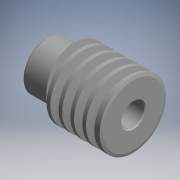
# Autodesk Inventor part: SW2-R1_On
Saved by Autodesk Inventor 2017.3 (Build 213256000, 256)
## iProperties
Part Number: SW2-R1_On
Material: Generic
Catalog Web Link: www.cadenas.de
Description: Worms, Worm Gears (SW)1-
Vendor: KHK
Document SubType Name: Modeling
Designer: partserver
Manufacturer: KHK
Mass: 24.6857 g
Surface Area: 108.891 cm^2
Volume: 24.6857 cm^3
Density: 1 g/cm^3
Appearance: PSOLRGB-192-192-192
Category: PARTsolutions
Company: KHK
Title: SW2-R1
Author: Cadenas PARTsolutions
PSOL_IDENT_0: {$CADENAS_DATA\23d-libs\khk\worms_worms_gears\ww_gears_sw.prj},178 {VTYP=3D},{NB=SW2-R1_On},{LINA=SW
PSOL_IDENT_1: 2-R1},{NN=Worms, Worm Gears (SW)1},{DATE=10.04.2020 06:07:44},{GEOMDATE=25.03.2019 13:28:29},{VERSIO
PSOL_IDENT_2: N=},{LINEID=120},{WBVAR=TOOTH},{WBNUMERIC=}  {NB=SW2-R1_On},{LINA=SW2-R1},{KT=DUMMY},{CN=SW2-R1},{NM=
PSOL_IDENT_3: 2.00},{NS=1},{LA=3.70},{HT=R},{SH=W1},{L=12},{M=25},{N=31},{O=35},{P=32},{Q=14},{Q1=0},{R=46},{K=0},
PSOL_IDENT_4: {KD=0.0},{SCS=0},{S=0},{WMF=W1002.WMF},{NDM=0},{KDM=0.000},{X=0.5},{Y=0.5},{H1=16.000},{AN=14.931},{
PSOL_IDENT_5: U=16},{COM1=1,'Only selection gear',201,'BG2-20R1',20,'CG2-20R1',30,'CG2-30R1',40,'CG2-40R1',50,'CG2
PSOL_IDENT_6: -50R1'},{XX=1},{TOOTH=On},{POINT=2.200}
NB: SW2-R1_On
NN: Worms, Worm Gears (SW)1
NBSYN: $CN._$TOOTH.
LINA: SW2-R1
CATALOG: KHK
CN: SW2-R1
NM: 2
NS: 1
LA: 3.7
HT: R
SH: W1
L: 12
M: 25
N: 31
O: 35
P: 32
Q: 14
Q1: 0
R: 46
K: 0
KD: 0
SCS: 0
S: 0
TOOTH: On
POINT: 2.2
SUPPLIER: KHK
ARTICLENO: SW2-R1_On
BOMINFO: SW2-R1
CREATOR: CADENAS GmbH
Autodesk Inventor part; units mm, degrees
sketch "Sketch_1" plane through (0, 0, 0) normal (0, 0, 1) x (1, 0, 0)
  line L0 (46, 0) -> (0, 0)
  line L1 (0, 6.5) -> (0.5, 6)
  line L2 (0.5, 6) -> (45.5, 6)
  line L3 (45.5, 6) -> (46, 6.5)
  line L4 (46, 6.5) -> (46, 12)
  line L5 (46, 12) -> (45.5, 12.5)
  line L6 (45.5, 12.5) -> (32, 12.5)
  line L7 (32, 12.5) -> (32, 16)
  line L8 (32, 16) -> (31.6, 17.5)
  line L9 (31.6, 17.5) -> (0.4, 17.5)
  line L10 (0.4, 17.5) -> (0, 16)
  line L11 (0, 16) -> (0, 6.5)
  constraints: 24 end point
revolve "Revolution1" add sketch "Sketch_1" angle 360 about axis through (46, 0, 0) along (1, 0, 0)
sketch "Sketch_18" plane through (0, 0, 0) normal (0, 0, 1) x (1, 0, 0)
  line L0 (5.6468, 0.1621) -> (3.14, 0)
  line L1 (0.0739, 20.8456) -> (2.3385, 12.3941)
  line L2 (2.3385, 12.3941) -> (4.8505, 12.3941)
  line L3 (4.8505, 12.3941) -> (5.6213, 21.2043)
  line L4 (5.6213, 21.2043) -> (0.0739, 20.8456)
  constraints: 10 end point
revolve "Revolution2" cut sketch "Sketch_18" angle 360 about axis through (5.6468, 0.1621, 0) along (0.9979, 0.0645, 0)
pattern_linear "Rectangular Pattern1" count 13 spacing 6.28 along (1, 0, 0) of "Revolution2"
sketch "Sketch_17" plane through (0, 0, 0) normal (0, 0, 1) x (1, 0, 0)
  line L0 (46, 0) -> (0, 0)
  line L1 (0, 9.25) -> (46, 9.25)
  line L2 (46, 9.25) -> (46, 12)
  line L3 (46, 12) -> (45.5, 12.5)
  line L4 (45.5, 12.5) -> (32, 12.5)
  line L5 (32, 12.5) -> (32, 13)
  line L6 (32, 13) -> (0, 13)
  line L7 (0, 13) -> (0, 9.25)
  constraints: 16 end point
revolve "Revolution3" add sketch "Sketch_17" angle 360 about axis through (46, 0, 0) along (1, 0, 0)
ref_plane "sw_XY" through (16.1197, 0, 0) normal (-1, 0, 0) x (0, 0, -1)
ref_plane "sw_YZ" through (16.1197, 0, 0) normal (0, 0, -1) x (0, -1, 0)
ref_plane "sw_ZX" through (16.1197, 0, 0) normal (0, -1, 0) x (-1, 0, 0)
body "Solid1"
